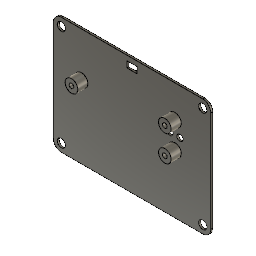
circuit_mount_plane v3 (Autodesk Fusion 360 design; units mm, degrees)
Autodesk Fusion 360 part; units mm, degrees
note: some values were not read from the file. Set by a fixed rule: which sketch regions a step uses.
sketch "Sketch1" plane through (0, 0, 0) normal (0, 1, 0) x (1, 0, 0)
  line L0 (0, 0) -> (70, 0)
  line L1 (70, 0) -> (70, -50)
  line L2 (70, -50) -> (0, -50)
  line L3 (0, -50) -> (0, 0)
  circle A0 centre (0, -50) radius 2
  circle A1 centre (0, 0) radius 2
  circle A2 centre (70, 0) radius 2
  circle A3 centre (70, -50) radius 2
  line L4 (0, 4) -> (70, 4)
  line L5 (74, 0) -> (74, -50)
  line L6 (70, -54) -> (0, -54)
  line L7 (-4, -50) -> (-4, 0)
  arc A4 (-4, -50) -> (0, -54) centre (0, -50) ccw
  arc A5 (0, 4) -> (-4, 0) centre (0, 0) ccw
  arc A6 (70, -54) -> (74, -50) centre (70, -50) ccw
  arc A7 (74, 0) -> (70, 4) centre (70, 0) ccw
  dimension "d1" = 70
  dimension "d2" = 50
  dimension "d3" = 4
  dimension "d4" = 4
  dimension "d5" = 4
  dimension "d6" = 4
  dimension "d8" = 4
  dimension "d9" = 4
  dimension "d10" = 4
  dimension "d11" = 4
  constraint horizontal L0
  constraint vertical L1
  constraint horizontal L2
  constraint vertical L3
  constraint coincident L0.start L3.end
  constraint coincident L2.end L3.start
  constraint coincident L0.end L1.start
  constraint coincident L1.end L2.start
  constraint parallel L0 L4
  constraint parallel L1 L5
  constraint parallel L2 L6
  constraint parallel L3 L7
  constraint tangent L6 A4
  constraint tangent L7 A4
  constraint tangent L4 A5
  constraint tangent L7 A5
  constraint tangent L5 A6
  constraint tangent L6 A6
  constraint tangent L4 A7
  constraint tangent L5 A7
  measures "d1" distance of L1.end L2.end
  measures "d2" distance of L0.start L2.end
  measures "d3" diameter of A0
  measures "d4" diameter of A1
  measures "d5" diameter of A2
  measures "d6" diameter of A3
  measures "d8" radius of A4
  measures "d9" radius of A5
  measures "d10" radius of A6
  measures "d11" radius of A7
extrude "Extrude1" add sketch "Sketch1" along normal blind 1 contours L0 L1 L2 L3 A0 A1 A2 A3 | L4 L5 L6 L7 A4 A5 A6 A7
sketch "Sketch2" plane through (0, 0, 0) normal (0, -1, 0) x (1, 0, 0)
  circle A0 centre (0, 0) radius 2
  circle A1 centre (0, 50) radius 2
  circle A2 centre (70, 0) radius 2
  circle A3 centre (70, 50) radius 2
  arc A4 (74, 50) -> (70, 54) centre (70, 50) ccw
  line L0 (70, 54) -> (0, 54)
  arc A5 (0, 54) -> (-4, 50) centre (0, 50) ccw
  line L1 (-4, 50) -> (-4, 0)
  arc A6 (-4, 0) -> (0, -4) centre (0, 0) ccw
  line L2 (0, -4) -> (70, -4)
  arc A7 (70, -4) -> (74, 0) centre (70, 0) ccw
  line L3 (74, 0) -> (74, 50)
  line L4 (10, 54) -> (10, -4)
  line L5 (56.228, 54) -> (56.228, -4)
  circle A8 centre (10, 32.046) radius 1.15
  circle A9 centre (56.228, 38.142) radius 1.15
  circle A10 centre (56.228, 25.188) radius 1.15
  line L6 (10, 45) -> (56.228, 45)
  line L7 (56.228, 45) -> (56.228, 5)
  line L8 (56.228, 5) -> (10, 5)
  line L9 (10, 5) -> (10, 45)
  line L10 (10, 25) -> (-4, 25)
  circle A11 centre (10, 32.046) radius 3.15
  circle A12 centre (56.228, 38.142) radius 3.15
  circle A13 centre (56.228, 25.188) radius 3.15
  line L11 (56.228, 38.142) -> (56.228, 25.188)
  circle A14 centre (53.728, 31.665) radius 1.5
  circle A15 centre (58.728, 31.665) radius 1.5
  line L12 (0, 50) -> (70, 50)
  line L13 (32.5, 51.5) -> (37.5, 51.5)
  line L14 (37.5, 51.5) -> (37.5, 48.5)
  line L15 (37.5, 48.5) -> (32.5, 48.5)
  line L16 (32.5, 48.5) -> (32.5, 51.5)
  line L17 (32.5, 51.5) -> (37.5, 48.5)
  line L18 (32.5, 48.5) -> (37.5, 51.5)
  line L19 (53.728, 31.665) -> (58.728, 31.665)
  point P0 (35, 50)
  point P1 (35, 50)
  point P2 (56.228, 31.665)
  point P3 (56.228, 31.665)
  dimension "d15" = 10
  dimension "d16" = 46.228
  dimension "d18" = 6.096
  dimension "d19" = 12.954
  dimension "d20" = 6.858
  dimension "d21" = 2.3
  dimension "d22" = 2.3
  dimension "d23" = 2.3
  dimension "d24" = 40
  dimension "d25" = 90
  dimension "d26" = 2
  dimension "d27" = 2
  dimension "d28" = 2
  dimension "d32" = 3
  dimension "d33" = 3
  dimension "d34" = 5
  dimension "d40" = 3
  dimension "d41" = 5
  constraint coincident L0 L4.start
  constraint coincident L2 L4.end
  constraint perpendicular L2 L4
  constraint coincident L0 L5.start
  constraint coincident L2 L5.end
  constraint perpendicular L2 L5
  constraint coincident L4 A8.centre
  constraint coincident L5 A9.centre
  constraint coincident L5 A10.centre
  constraint horizontal L6
  constraint vertical L7
  constraint horizontal L8
  constraint vertical L9
  constraint coincident L5 L7.end
  constraint coincident L4 L6.start
  constraint midpoint L9 L10.start
  constraint midpoint L1 L10.end
  constraint coincident A9.centre A12.centre
  constraint coincident A10.centre A13.centre
  constraint coincident A1.centre A5.centre
  constraint coincident A3.centre A4.centre
  constraint horizontal L13
  constraint vertical L14
  constraint horizontal L15
  constraint vertical L16
  constraint midpoint L12 P1
  constraint midpoint L17 P1
  constraint coincident P1 P0
  constraint coincident A14.centre L19.start
  constraint coincident A15.centre L19.end
  constraint horizontal L19
  constraint midpoint L19 P3
  constraint midpoint L11 P3
  constraint coincident P3 P2
  measures "d15" distance of A1.centre L4
  measures "d16" distance of L4 L5
  measures "d18" vertical distance of A8.centre A9.centre
  measures "d19" distance of A9.centre A10.centre
  measures "d20" distance of A9.centre L6
  measures "d21" diameter of A8
  measures "d22" diameter of A9
  measures "d23" diameter of A10
  measures "d24" distance of L6 L8
  measures "d25" angle of L1 L10
  measures "d32" diameter of A14
  measures "d33" diameter of A15
  measures "d34" distance of A14.centre A15.centre
  measures "d40" distance of L13.start L15.end
  measures "d41" distance of L13.start L13.end
extrude "Extrude2" add sketch "Sketch2" along normal blind 5 contours L5 A9 L7 A12 L11 | L5 A9 L7 A12 L11 | L5 A10 L7 A13 L11 | L5 A10 L7 A13 L11 | L4 A8 L9 A11 | L4 A8 L9 A11
extrude "Extrude3" cut sketch "Sketch2" against normal blind 5 contours L12 L14 L17 | L12 L14 L18 | L12 L16 L17 | L12 L16 L18 | L15 L17 L18 | L13 L17 L18 | A14 | A15
